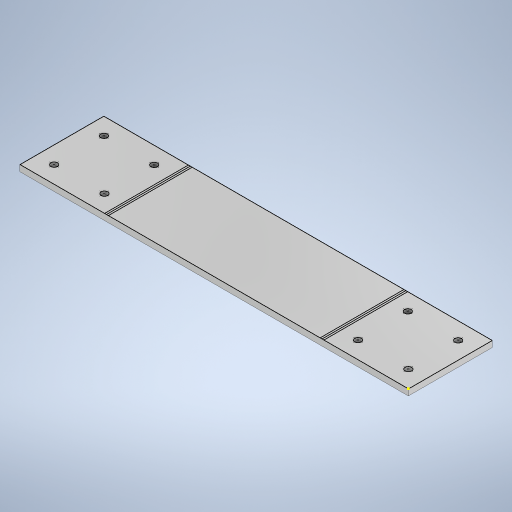
# Autodesk Inventor part: axis_3_bottom_frame(middle)
Saved by Autodesk Inventor 2024.2 (Build 282272000, 272)
## iProperties
Created: 2023-12-25
Part Number: axis_3_bottom_frame(middle)
Material: Aluminum 6061-AHC
Document SubType Name: Modeling
Designer: chanh
Density: 2.7 g/cm^3
Appearance: Aluminum - Dark
Author: chanh
Autodesk Inventor part; units mm, degrees
ref_plane "YZ Plane" through (0, 0, 0) normal (1, 0, 0) x (0, 1, 0)
ref_plane "XZ Plane" through (0, 0, 0) normal (0, 1, 0) x (-1, 0, 0)
ref_plane "XY Plane" through (0, 0, 0) normal (0, 0, 1) x (1, 0, 0)
sketch "Sketch1" plane through (0, 0, 0) normal (0, 1, 0) x (-1, 0, 0)
  line L0 (20.6396, 0) -> (20.6396, -20)
  line L1 (72.0989, -20) -> (72.0989, 0)
  circle A0 centre (88.6436, -4.0565) radius 0.7835
  circle A1 centre (4.095, -4.0565) radius 0.7835
  circle A2 centre (76.6436, -4.0565) radius 0.7835
  circle A3 centre (16.095, -4.0565) radius 0.7835
  circle A4 centre (88.6436, -15.9435) radius 0.7835
  circle A5 centre (4.095, -15.9435) radius 0.7835
  circle A6 centre (76.6436, -15.9435) radius 0.7835
  circle A7 centre (16.095, -15.9435) radius 0.7835
  line L2 (0, -20) -> (0, 0)
  line L3 (92.7386, -20) -> (0, -20)
  line L4 (0, 0) -> (92.7386, 0)
  line L5 (92.7386, 0) -> (92.7386, -20)
  line L6 (72.5486, 0) -> (72.5486, -20)
  line L7 (71.6493, -20) -> (71.6493, 0)
  line L8 (21.0893, 0) -> (21.0893, -20)
  line L9 (20.19, -20) -> (20.19, 0)
  point P0 (0, 0)
  constraints: 20 end point, 12 point on line, 8 centre point, 8 vertical, 2 horizontal, 33 other
extrude "Extrusion1" add sketch "Sketch1" against normal blind 1.5
body "Solid1"
